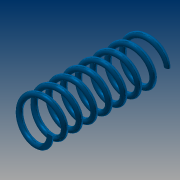
# Autodesk Inventor part: SPRING
Saved by Autodesk Inventor 2014 (Build 180170000, 170)
## iProperties
Created: 2021-03-21
Part Number: SPRING
Material: Stainless Steel
Document SubType Name: Modeling
Designer: Think Station
Density: 8.08 g/cm^3
Appearance: Semi-Polished(1)
Mass: 138.205 g
Surface Area: 138.478 cm^2
Volume: 17.1045 cm^3
Author: Think Station
Autodesk Inventor part; units mm, degrees
ref_plane "YZ Plane" through (0, 0, 0) normal (1, 0, 0) x (0, 1, 0)
ref_plane "XZ Plane" through (0, 0, 0) normal (0, 1, 0) x (-1, 0, 0)
ref_plane "XY Plane" through (0, 0, 0) normal (0, 0, 1) x (1, 0, 0)
sketch "Sketch1" plane through (0, 0, 0) normal (0, 1, 0) x (-1, 0, 0)
  circle A0 centre (0, 0) radius 20
  dimension "d0" = 40
  constraints: 1 centre point, 1 coincident
  measures "d0" diameter of A0
extrude "Extrusion1" add sketch "Sketch1" along normal blind 110
sketch "Sketch2" plane through (0, 0, 0) normal (0, 0, 1) x (1, 0, 0)
  line L0 (20, 110) -> (-20, 110) construction
  line L1 (0, 0) -> (0, 110) construction
  circle A0 centre (17.5, 0) radius 2.5
  line L2 (-20, 0) -> (20, 0) projected
  line L3 (0, 110) -> (20, 110) construction
  line L4 (20, 110) -> (20, 0) construction
  dimension "d3" = 5
  dimension "d4" = 17.5
  dimension "d13" = 110
  constraints: 6 end point, 1 centre point, 1 collinear, 1 midpoint, 1 perpendicular, 1 point on line
  measures "d3" diameter of A0
  measures "d4" distance of A0.centre L1.start
  measures "d13" distance of L0.start L2.end
coil "Coil1" sketch "Sketch2" operation intersect axis through (0, 0, 0) along (0, 1, 0) pitch 13.75 turns 8 hand right
equation "\"d6\" = d13"
body "Solid1"
